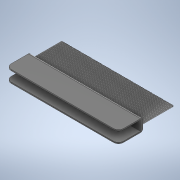
# Autodesk Inventor part: Kabeldurchführung
Saved by Autodesk Inventor 2021 (Build 250183000, 183)
## iProperties
Created: 2021-05-14
Part Number: Kabeldurchführung
Material: Generisch
Document SubType Name: Modeling
Designer: Sebastian Seewald
Density: 1 g/cm^3
Appearance: Vorgabe
Author: Sebastian Seewald
Autodesk Inventor part; units mm, degrees
ref_plane "YZ Plane" through (0, 0, 0) normal (1, 0, 0) x (0, 1, 0)
ref_plane "XZ Plane" through (0, 0, 0) normal (0, 1, 0) x (-1, 0, 0)
ref_plane "XY Plane" through (0, 0, 0) normal (0, 0, 1) x (1, 0, 0)
sketch "Skizze1" plane through (0, 0, 0) normal (0, 0, 1) x (1, 0, 0)
  line L0 (-23, 2.5) -> (23, 2.5)
  line L1 (23, 2.5) -> (23, -2.5)
  line L2 (23, -2.5) -> (-23, -2.5)
  line L3 (-23, -2.5) -> (-23, 2.5)
  point P0 (0, 0)
  dimension "d0" = 5
  dimension "d1" = 46
  dimension "d2" = 23
  dimension "d3" = 2.5
  constraints: 8 end point, 2 parallel, 1 horizontal, 1 perpendicular
  measures "d0" distance between parallel lines of L2 L0
  measures "d1" distance of L0.start L0.end
  measures "d2" distance from line of point (0, 0) L1
  measures "d3" distance from line of point (0, 0) L2
extrude "Extrusion1" add sketch "Skizze1" along normal blind 10
sketch "Skizze2" plane through (0, 0, 10) normal (0, 0, 1) x (1, 0, 0)
  line L0 (-23, 2.5) -> (-23, -2.5) projected
  line L1 (23, -2.5) -> (23, 2.5) projected
  line L2 (-23, 2) -> (23, 2)
  line L3 (23, 2) -> (23, -2)
  line L4 (23, -2) -> (-23, -2)
  line L5 (-23, -2) -> (-23, 2)
  line L6 (-23, -2.5) -> (23, -2.5) projected
  point P0 (0, 0)
  dimension "d6" = 4
  dimension "d7" = 0.5
  constraints: 8 end point, 2 parallel, 2 point on line, 1 horizontal, 1 perpendicular
  measures "d6" distance between parallel lines of L4 L2
  measures "d7" distance between parallel lines of L6 L4
extrude "Extrusion2" cut sketch "Skizze2" against normal blind 9 contours L2 L1 L4 L0
fillet "Rundung1" radius 2 4 edges at (-23, 2.25, 10) (-23, -2.25, 10) (23, -2.25, 10) (23, 2.25, 10)
sketch "Skizze3" plane through (0, 0, 0) normal (0, 0, -1) x (-1, 0, 0)
  circle A0 centre (22.9, -0.2) radius 0.1
  line L0 (23, 2.5) -> (23, -2.5) projected
  point P0 (0, 0)
  dimension "d11" = 0.2
  dimension "d12" = 0.2
  dimension "d13" = 0.1
  constraints: 1 centre point
  measures "d11" diameter of A0
  measures "d12" vertical distance of point (0, 0) A0.centre
  measures "d13" distance from line of A0.centre L0
extrude "Extrusion3" add sketch "Skizze3" along normal blind 12.65
pattern_linear "Rechteckige Anordnung1" count 153 spacing 0.3 along (1, 0, 0) count 2 spacing 0.4 along (0, 1, 0) of "Extrusion3"
fillet "Rundung2" radius 1 2 edges at (0, -2.5, 0) (0, 2.5, 0)
